Autodesk Inventor part; units mm, degrees
(part 2 of 2)
sketch "スケッチ14" plane through (-202, -25, 10) normal (-1, 0, 0) x (0, 0, 1)
  line L0 (48, 4) -> (0, 4) projected
  line L1 (0, 0) -> (0, 4) projected
  line L2 (0, 0) -> (52, 0) projected
  line L3 (52, 50) -> (52, 0) projected
  line L4 (0, 50) -> (52, 50) projected
  line L5 (0, 46) -> (0, 50) projected
  line L6 (0, 46) -> (48, 46) projected
  line L7 (48, 46) -> (48, 4) projected
  line L8 (-13.92, 46) -> (-6.08, 46) projected
  line L9 (-6.08, 46) -> (-10, 32.2801) projected
  line L10 (-10, 32.2801) -> (-13.92, 46) projected
  line L11 (-16, 38.7199) -> (-12.08, 25) projected
  line L12 (-12.08, 25) -> (-16, 11.2801) projected
  line L13 (-16, 11.2801) -> (-16, 38.7199) projected
  line L14 (-13.92, 4) -> (-10, 17.7199) projected
  line L15 (-10, 17.7199) -> (-6.08, 4) projected
  line L16 (-6.08, 4) -> (-13.92, 4) projected
  line L17 (-4, 11.2801) -> (-7.92, 25) projected
  line L18 (-7.92, 25) -> (-4, 38.7199) projected
  line L19 (-4, 38.7199) -> (-4, 11.2801) projected
  line L20 (-20, 0) -> (0, 0) projected
  line L21 (0, 0) -> (0, 50) projected
  line L22 (0, 50) -> (-20, 50) projected
  line L23 (-20, 50) -> (-20, 0) projected
  line L24 (48, 46) -> (27.8284, 46) projected
  line L25 (44.481, 46) -> (24, 27.4342)
  line L26 (24, 27.4342) -> (4.2197, 46)
  line L27 (0, 46) -> (22.1716, 46) projected
  line L28 (48, 46) -> (24.3744, 24.5837)
  line L29 (27.8284, 4) -> (48, 4) projected
  line L30 (0, 27.7082) -> (0, 46) projected
  line L31 (48, 4) -> (0, 46)
  line L32 (48, 4) -> (48, 46) projected
  line L33 (48, 25) -> (37.9142, 25)
  point P0 (-10, 25)
  dimension "d178" = 2
  constraints: 10 end point, 2 point on line, 1 horizontal, 1 midpoint, 1 parallel
  measures "d178" angle of L31 L26
sketch "スケッチ15" plane through (-202, -25, 10) normal (-1, 0, 0) x (0, 0, 1)
  line L0 (48, 4) -> (0, 4) projected
  line L1 (0, 0) -> (0, 4) projected
  line L2 (0, 0) -> (52, 0) projected
  line L3 (52, 50) -> (52, 0) projected
  line L4 (0, 50) -> (52, 50) projected
  line L5 (0, 46) -> (0, 50) projected
  line L6 (0, 46) -> (48, 46) projected
  line L7 (48, 46) -> (48, 4) projected
  line L8 (48, 46) -> (27.8284, 46) projected
  line L9 (44.3624, 46) -> (0, 5.9989)
  line L10 (0, 4) -> (0, 22.2918) projected
  line L11 (48, 45.1716) -> (48, 27) projected
  line L12 (48, 43.894) -> (3.7564, 4)
  line L13 (0, 4) -> (22.1716, 4) projected
  line L14 (48, 4) -> (48, 46) projected
  line L15 (48, 25) -> (41.7662, 25)
  line L16 (44.3624, 4) -> (0, 44.0011)
  line L17 (48, 6.106) -> (3.7564, 46)
  line L18 (18.8547, 27) -> (0, 27)
  line L19 (0, 27) -> (0, 23)
  line L20 (0, 6.7082) -> (0, 43.2918) projected
  line L21 (0, 23) -> (18.8547, 23)
  point P0 (-10, 25)
  dimension "d179" = 4
  dimension "d180" = 4
  constraints: 16 end point, 7 point on line, 4 symmetric about line, 2 horizontal, 1 midpoint, 1 parallel, 1 perpendicular
  measures "d179" distance between parallel lines of L12 L9
  measures "d180" distance of L18.end L19.end
sketch "スケッチ16" plane through (250, -25, 10) normal (0, 0, 1) x (1, 0, 0)
  line L0 (-97.1716, 4) -> (-102.8284, 4) projected
  line L1 (-97.1716, 0) -> (-97.1716, 4) projected
  line L2 (-52.8284, 0) -> (-97.1716, 0) projected
  line L3 (-52.8284, 0) -> (-52.8284, 4) projected
  line L4 (-50, 4) -> (-52.8284, 4) projected
  line L5 (-50, 4) -> (-50, 0) projected
  line L6 (0, 0) -> (-50, 0) projected
  line L7 (0, 50) -> (0, 0) projected
  line L8 (-50, 50) -> (0, 50) projected
  line L9 (-50, 50) -> (-50, 46) projected
  line L10 (-50, 46) -> (-52.8284, 46) projected
  line L11 (-52.8284, 46) -> (-52.8284, 50) projected
  line L12 (-97.1716, 50) -> (-52.8284, 50) projected
  line L13 (-97.1716, 46) -> (-97.1716, 50) projected
  line L14 (-97.1716, 46) -> (-102.8284, 46) projected
  line L15 (-102.8284, 46) -> (-102.8284, 50) projected
  line L16 (-147.1716, 50) -> (-102.8284, 50) projected
  line L17 (-147.1716, 46) -> (-147.1716, 50) projected
  line L18 (-147.1716, 46) -> (-152.8284, 46) projected
  line L19 (-152.8284, 46) -> (-152.8284, 50) projected
  line L20 (-197.1716, 50) -> (-152.8284, 50) projected
  line L21 (-197.1716, 46) -> (-197.1716, 50) projected
  line L22 (-197.1716, 46) -> (-202.8284, 46) projected
  line L23 (-202.8284, 46) -> (-202.8284, 50) projected
  line L24 (-247.1716, 50) -> (-202.8284, 50) projected
  line L25 (-247.1716, 46) -> (-247.1716, 50) projected
  line L26 (-247.1716, 46) -> (-252.8284, 46) projected
  line L27 (-252.8284, 46) -> (-252.8284, 50) projected
  line L28 (-297.1716, 50) -> (-252.8284, 50) projected
  line L29 (-297.1716, 46) -> (-297.1716, 50) projected
  line L30 (-297.1716, 46) -> (-302.8284, 46) projected
  line L31 (-302.8284, 46) -> (-302.8284, 50) projected
  line L32 (-347.1716, 50) -> (-302.8284, 50) projected
  line L33 (-347.1716, 46) -> (-347.1716, 50) projected
  line L34 (-347.1716, 46) -> (-352.8284, 46) projected
  line L35 (-352.8284, 46) -> (-352.8284, 50) projected
  line L36 (-397.1716, 50) -> (-352.8284, 50) projected
  line L37 (-397.1716, 46) -> (-397.1716, 50) projected
  line L38 (-397.1716, 46) -> (-402.8284, 46) projected
  line L39 (-402.8284, 46) -> (-402.8284, 50) projected
  line L40 (-447.1716, 50) -> (-402.8284, 50) projected
  line L41 (-447.1716, 46) -> (-447.1716, 50) projected
  line L42 (-447.1716, 46) -> (-452, 46) projected
  line L43 (-452, 46) -> (-452, 50) projected
  line L44 (-500, 50) -> (-452, 50) projected
  line L45 (-500, 0) -> (-500, 50) projected
  line L46 (-452, 0) -> (-500, 0) projected
  line L47 (-452, 0) -> (-452, 4) projected
  line L48 (-447.1716, 4) -> (-452, 4) projected
  line L49 (-447.1716, 0) -> (-447.1716, 4) projected
  line L50 (-402.8284, 0) -> (-447.1716, 0) projected
  line L51 (-402.8284, 0) -> (-402.8284, 4) projected
  line L52 (-397.1716, 4) -> (-402.8284, 4) projected
  line L53 (-397.1716, 0) -> (-397.1716, 4) projected
  line L54 (-352.8284, 0) -> (-397.1716, 0) projected
  line L55 (-352.8284, 0) -> (-352.8284, 4) projected
  line L56 (-347.1716, 4) -> (-352.8284, 4) projected
  line L57 (-347.1716, 0) -> (-347.1716, 4) projected
  line L58 (-302.8284, 0) -> (-347.1716, 0) projected
  line L59 (-302.8284, 0) -> (-302.8284, 4) projected
  line L60 (-297.1716, 4) -> (-302.8284, 4) projected
  line L61 (-297.1716, 0) -> (-297.1716, 4) projected
  line L62 (-252.8284, 0) -> (-297.1716, 0) projected
  line L63 (-252.8284, 0) -> (-252.8284, 4) projected
  line L64 (-247.1716, 4) -> (-252.8284, 4) projected
  line L65 (-247.1716, 0) -> (-247.1716, 4) projected
  line L66 (-202.8284, 0) -> (-247.1716, 0) projected
  line L67 (-202.8284, 0) -> (-202.8284, 4) projected
  line L68 (-197.1716, 4) -> (-202.8284, 4) projected
  line L69 (-197.1716, 0) -> (-197.1716, 4) projected
  line L70 (-152.8284, 0) -> (-197.1716, 0) projected
  line L71 (-152.8284, 0) -> (-152.8284, 4) projected
  line L72 (-147.1716, 4) -> (-152.8284, 4) projected
  line L73 (-147.1716, 0) -> (-147.1716, 4) projected
  line L74 (-102.8284, 0) -> (-147.1716, 0) projected
  line L75 (-102.8284, 0) -> (-102.8284, 4) projected
  line L76 (-152, 6.7082) -> (-172.0338, 25) projected
  line L77 (-172.0338, 25) -> (-152, 43.2918) projected
  line L78 (-152, 43.2918) -> (-152, 6.7082) projected
  line L79 (-177.9662, 25) -> (-198, 6.7082) projected
  line L80 (-198, 6.7082) -> (-198, 43.2918) projected
  line L81 (-198, 43.2918) -> (-177.9662, 25) projected
  line L82 (-154.9662, 4) -> (-195.0338, 4) projected
  line L83 (-195.0338, 4) -> (-175, 22.2918) projected
  line L84 (-175, 22.2918) -> (-154.9662, 4) projected
  line L85 (-154.9662, 46) -> (-175, 27.7082) projected
  line L86 (-175, 27.7082) -> (-195.0338, 46) projected
  line L87 (-195.0338, 46) -> (-154.9662, 46) projected
  line L88 (-227.9662, 25) -> (-248, 6.7082) projected
  line L89 (-248, 6.7082) -> (-248, 43.2918) projected
  line L90 (-248, 43.2918) -> (-227.9662, 25) projected
  line L91 (-202, 6.7082) -> (-222.0338, 25) projected
  line L92 (-222.0338, 25) -> (-202, 43.2918) projected
  line L93 (-202, 43.2918) -> (-202, 6.7082) projected
  line L94 (-204.9662, 4) -> (-245.0338, 4) projected
  line L95 (-245.0338, 4) -> (-225, 22.2918) projected
  line L96 (-225, 22.2918) -> (-204.9662, 4) projected
  line L97 (-204.9662, 46) -> (-225, 27.7082) projected
  line L98 (-225, 27.7082) -> (-245.0338, 46) projected
  line L99 (-245.0338, 46) -> (-204.9662, 46) projected
  line L100 (-252, 6.7082) -> (-272.0338, 25) projected
  line L101 (-272.0338, 25) -> (-252, 43.2918) projected
  line L102 (-252, 6.7082) -> (-252, 43.2918) projected
  line L103 (-345.0338, 4) -> (-325, 22.2918) projected
  line L104 (-325, 22.2918) -> (-304.9662, 4) projected
  line L105 (-345.0338, 4) -> (-304.9662, 4) projected
  line L106 (-254.9662, 46) -> (-275, 27.7082) projected
  line L107 (-275, 27.7082) -> (-295.0338, 46) projected
  line L108 (-254.9662, 46) -> (-295.0338, 46) projected
  line L109 (-304.9662, 46) -> (-345.0338, 46) projected
  line L110 (-304.9662, 46) -> (-325, 27.7082) projected
  line L111 (-325, 27.7082) -> (-345.0338, 46) projected
  line L112 (-354.9662, 46) -> (-375, 27.7082) projected
  line L113 (-375, 27.7082) -> (-395.0338, 46) projected
  line L114 (-354.9662, 46) -> (-395.0338, 46) projected
  line L115 (-295.0338, 4) -> (-254.9662, 4) projected
  line L116 (-295.0338, 4) -> (-275, 22.2918) projected
  line L117 (-275, 22.2918) -> (-254.9662, 4) projected
  line L118 (-395.0338, 4) -> (-354.9662, 4) projected
  line L119 (-395.0338, 4) -> (-375, 22.2918) projected
  line L120 (-375, 22.2918) -> (-354.9662, 4) projected
  line L121 (-445.0338, 4) -> (-425, 22.2918) projected
  line L122 (-425, 22.2918) -> (-404.9662, 4) projected
  line L123 (-445.0338, 4) -> (-404.9662, 4) projected
  line L124 (-404.9662, 46) -> (-445.0338, 46) projected
  line L125 (-404.9662, 46) -> (-425, 27.7082) projected
  line L126 (-425, 27.7082) -> (-445.0338, 46) projected
  line L127 (-322.0338, 25) -> (-302, 43.2918) projected
  line L128 (-302, 43.2918) -> (-302, 6.7082) projected
  line L129 (-302, 6.7082) -> (-322.0338, 25) projected
  line L130 (-298, 43.2918) -> (-277.9662, 25) projected
  line L131 (-277.9662, 25) -> (-298, 6.7082) projected
  line L132 (-298, 6.7082) -> (-298, 43.2918) projected
  line L133 (-372.0338, 25) -> (-352, 43.2918) projected
  line L134 (-352, 43.2918) -> (-352, 6.7082) projected
  line L135 (-352, 6.7082) -> (-372.0338, 25) projected
  line L136 (-348, 43.2918) -> (-327.9662, 25) projected
  line L137 (-327.9662, 25) -> (-348, 6.7082) projected
  line L138 (-348, 6.7082) -> (-348, 43.2918) projected
  line L139 (-452, 4.8284) -> (-471.6499, 24.4784) projected
  line L140 (-471.6499, 24.4784) -> (-452, 43.2351) projected
  line L141 (-452, 4.8284) -> (-452, 43.2351) projected
  line L142 (-456.8284, 4) -> (-493.1034, 4) projected
  line L143 (-493.1034, 4) -> (-474.5441, 21.7157) projected
  line L144 (-474.5441, 21.7157) -> (-456.8284, 4) projected
  line L145 (-496, 6.7649) -> (-496, 43.1716) projected
  line L146 (-496, 43.1716) -> (-477.3733, 24.5449) projected
  line L147 (-477.3733, 24.5449) -> (-496, 6.7649) projected
  line L148 (-454.8966, 46) -> (-474.4791, 27.3075) projected
  line L149 (-474.4791, 27.3075) -> (-493.1716, 46) projected
  line L150 (-493.1716, 46) -> (-454.8966, 46) projected
  line L151 (-448, 43.2918) -> (-427.9662, 25) projected
  line L152 (-427.9662, 25) -> (-448, 6.7082) projected
  line L153 (-448, 6.7082) -> (-448, 43.2918) projected
  line L154 (-422.0338, 25) -> (-402, 43.2918) projected
  line L155 (-402, 43.2918) -> (-402, 6.7082) projected
  line L156 (-402, 6.7082) -> (-422.0338, 25) projected
  line L157 (-398, 43.2918) -> (-377.9662, 25) projected
  line L158 (-377.9662, 25) -> (-398, 6.7082) projected
  line L159 (-398, 6.7082) -> (-398, 43.2918) projected
  line L160 (-104.9662, 4) -> (-145.0338, 4) projected
  line L161 (-145.0338, 4) -> (-125, 22.2918) projected
  line L162 (-125, 22.2918) -> (-104.9662, 4) projected
  line L163 (-104.9662, 46) -> (-125, 27.7082) projected
  line L164 (-125, 27.7082) -> (-145.0338, 46) projected
  line L165 (-145.0338, 46) -> (-104.9662, 46) projected
  line L166 (-127.9662, 25) -> (-148, 6.7082) projected
  line L167 (-148, 6.7082) -> (-148, 43.2918) projected
  line L168 (-148, 43.2918) -> (-127.9662, 25) projected
  line L169 (-102, 6.7082) -> (-122.0338, 25) projected
  line L170 (-122.0338, 25) -> (-102, 43.2918) projected
  line L171 (-102, 43.2918) -> (-102, 6.7082) projected
  line L172 (-54.9662, 46) -> (-75, 27.7082) projected
  line L173 (-75, 27.7082) -> (-95.0338, 46) projected
  line L174 (-95.0338, 46) -> (-54.9662, 46) projected
  line L175 (-54.9662, 4) -> (-95.0338, 4) projected
  line L176 (-95.0338, 4) -> (-75, 22.2918) projected
  line L177 (-75, 22.2918) -> (-54.9662, 4) projected
  line L178 (-77.9662, 25) -> (-98, 6.7082) projected
  line L179 (-98, 6.7082) -> (-98, 43.2918) projected
  line L180 (-98, 43.2918) -> (-77.9662, 25) projected
  line L181 (-52, 6.7082) -> (-72.0338, 25) projected
  line L182 (-72.0338, 25) -> (-52, 43.2918) projected
  line L183 (-52, 43.2918) -> (-52, 6.7082) projected
  line L184 (-4, 6.7649) -> (-22.6267, 24.5449) projected
  line L185 (-22.6267, 24.5449) -> (-4, 43.1716) projected
  line L186 (-4, 43.1716) -> (-4, 6.7649) projected
  line L187 (-6.8284, 46) -> (-25.5209, 27.3075) projected
  line L188 (-25.5209, 27.3075) -> (-45.1034, 46) projected
  line L189 (-45.1034, 46) -> (-6.8284, 46) projected
  line L190 (-43.1716, 4) -> (-25.4559, 21.7157) projected
  line L191 (-25.4559, 21.7157) -> (-6.8966, 4) projected
  line L192 (-6.8966, 4) -> (-43.1716, 4) projected
  line L193 (-48, 43.2351) -> (-28.3501, 24.4784) projected
  line L194 (-28.3501, 24.4784) -> (-48, 4.8284) projected
  line L195 (-48, 4.8284) -> (-48, 43.2351) projected
  line L196 (-452, 4.8284) -> (-452, 43.2351) projected
  line L197 (-452, 27.0005) -> (-448, 27.0005)
  line L198 (-448, 27.0005) -> (-448, 23.0005)
  line L199 (-448, 23.0005) -> (-452, 23.0005)
  line L200 (-452, 23.0005) -> (-452, 27.0005)
  point P0 (-250, 25)
  dimension "d181" = 4
  dimension "d182" = 4
  constraints: 8 end point, 2 parallel, 1 horizontal, 1 perpendicular, 1 point on line
  measures "d181" distance of L198.end L199.end
  measures "d182" distance of L197.end L198.end
extrude "押し出し24" add sketch "スケッチ16" along normal blind 48 contours L141 L197 L153 L199
pattern_linear "矩形状パターン3" count 9 spacing 50 along (1, 0, 0) of "押し出し24"
sketch "スケッチ17" plane through (250, -25, 10) normal (0, 0, 1) x (1, 0, 0)
  line L0 (-52, 27.0005) -> (-48, 27.0005) projected
  line L1 (-48, 27.0005) -> (-48, 43.2351) projected
  line L2 (-48, 43.2351) -> (-28.3501, 24.4784) projected
  line L3 (-28.3501, 24.4784) -> (-48, 4.8284) projected
  line L4 (-48, 4.8284) -> (-48, 23.0005) projected
  line L5 (-48, 23.0005) -> (-52, 23.0005) projected
  line L6 (-52, 23.0005) -> (-52, 6.7082) projected
  line L7 (-52, 6.7082) -> (-72.0338, 25) projected
  line L8 (-72.0338, 25) -> (-52, 43.2918) projected
  line L9 (-52, 43.2918) -> (-52, 27.0005) projected
  line L10 (-43.1716, 4) -> (-25.4559, 21.7157) projected
  line L11 (-25.4559, 21.7157) -> (-6.8966, 4) projected
  line L12 (-6.8966, 4) -> (-43.1716, 4) projected
  line L13 (-6.8284, 46) -> (-25.5209, 27.3075) projected
  line L14 (-25.5209, 27.3075) -> (-45.1034, 46) projected
  line L15 (-45.1034, 46) -> (-6.8284, 46) projected
  line L16 (-4, 6.7649) -> (-22.6267, 24.5449) projected
  line L17 (-22.6267, 24.5449) -> (-4, 43.1716) projected
  line L18 (-4, 43.1716) -> (-4, 6.7649) projected
  line L19 (-102, 27.0005) -> (-98, 27.0005) projected
  line L20 (-98, 27.0005) -> (-98, 43.2918) projected
  line L21 (-98, 43.2918) -> (-77.9662, 25) projected
  line L22 (-77.9662, 25) -> (-98, 6.7082) projected
  line L23 (-98, 6.7082) -> (-98, 23.0005) projected
  line L24 (-98, 23.0005) -> (-102, 23.0005) projected
  line L25 (-102, 23.0005) -> (-102, 6.7082) projected
  line L26 (-102, 6.7082) -> (-122.0338, 25) projected
  line L27 (-122.0338, 25) -> (-102, 43.2918) projected
  line L28 (-102, 43.2918) -> (-102, 27.0005) projected
  line L29 (-54.9662, 4) -> (-95.0338, 4) projected
  line L30 (-95.0338, 4) -> (-75, 22.2918) projected
  line L31 (-75, 22.2918) -> (-54.9662, 4) projected
  line L32 (-54.9662, 46) -> (-75, 27.7082) projected
  line L33 (-75, 27.7082) -> (-95.0338, 46) projected
  line L34 (-95.0338, 46) -> (-54.9662, 46) projected
  line L35 (-152, 27.0005) -> (-148, 27.0005) projected
  line L36 (-148, 27.0005) -> (-148, 43.2918) projected
  line L37 (-148, 43.2918) -> (-127.9662, 25) projected
  line L38 (-127.9662, 25) -> (-148, 6.7082) projected
  line L39 (-148, 6.7082) -> (-148, 23.0005) projected
  line L40 (-148, 23.0005) -> (-152, 23.0005) projected
  line L41 (-152, 23.0005) -> (-152, 6.7082) projected
  line L42 (-152, 6.7082) -> (-172.0338, 25) projected
  line L43 (-172.0338, 25) -> (-152, 43.2918) projected
  line L44 (-152, 43.2918) -> (-152, 27.0005) projected
  line L45 (-104.9662, 46) -> (-125, 27.7082) projected
  line L46 (-125, 27.7082) -> (-145.0338, 46) projected
  line L47 (-145.0338, 46) -> (-104.9662, 46) projected
  line L48 (-104.9662, 4) -> (-145.0338, 4) projected
  line L49 (-145.0338, 4) -> (-125, 22.2918) projected
  line L50 (-125, 22.2918) -> (-104.9662, 4) projected
  line L51 (-402, 27.0005) -> (-398, 27.0005) projected
  line L52 (-398, 27.0005) -> (-398, 43.2918) projected
  line L53 (-398, 43.2918) -> (-377.9662, 25) projected
  line L54 (-377.9662, 25) -> (-398, 6.7082) projected
  line L55 (-398, 6.7082) -> (-398, 23.0005) projected
  line L56 (-398, 23.0005) -> (-402, 23.0005) projected
  line L57 (-402, 23.0005) -> (-402, 6.7082) projected
  line L58 (-402, 6.7082) -> (-422.0338, 25) projected
  line L59 (-422.0338, 25) -> (-402, 43.2918) projected
  line L60 (-402, 43.2918) -> (-402, 27.0005) projected
  line L61 (-452, 27.0005) -> (-448, 27.0005) projected
  line L62 (-448, 27.0005) -> (-448, 43.2918) projected
  line L63 (-448, 43.2918) -> (-427.9662, 25) projected
  line L64 (-427.9662, 25) -> (-448, 6.7082) projected
  line L65 (-448, 6.7082) -> (-448, 23.0005) projected
  line L66 (-448, 23.0005) -> (-452, 23.0005) projected
  line L67 (-452, 4.8284) -> (-452, 23.0005) projected
  line L68 (-452, 4.8284) -> (-471.6499, 24.4784) projected
  line L69 (-471.6499, 24.4784) -> (-452, 43.2351) projected
  line L70 (-452, 27.0005) -> (-452, 43.2351) projected
  line L71 (-454.8966, 46) -> (-474.4791, 27.3075) projected
  line L72 (-474.4791, 27.3075) -> (-493.1716, 46) projected
  line L73 (-493.1716, 46) -> (-454.8966, 46) projected
  line L74 (-496, 6.7649) -> (-496, 43.1716) projected
  line L75 (-496, 43.1716) -> (-477.3733, 24.5449) projected
  line L76 (-477.3733, 24.5449) -> (-496, 6.7649) projected
  line L77 (-456.8284, 4) -> (-493.1034, 4) projected
  line L78 (-493.1034, 4) -> (-474.5441, 21.7157) projected
  line L79 (-474.5441, 21.7157) -> (-456.8284, 4) projected
  line L80 (-352, 27.0005) -> (-348, 27.0005) projected
  line L81 (-348, 27.0005) -> (-348, 43.2918) projected
  line L82 (-348, 43.2918) -> (-327.9662, 25) projected
  line L83 (-327.9662, 25) -> (-348, 6.7082) projected
  line L84 (-348, 6.7082) -> (-348, 23.0005) projected
  line L85 (-348, 23.0005) -> (-352, 23.0005) projected
  line L86 (-352, 23.0005) -> (-352, 6.7082) projected
  line L87 (-352, 6.7082) -> (-372.0338, 25) projected
  line L88 (-372.0338, 25) -> (-352, 43.2918) projected
  line L89 (-352, 43.2918) -> (-352, 27.0005) projected
  line L90 (-302, 27.0005) -> (-298, 27.0005) projected
  line L91 (-298, 27.0005) -> (-298, 43.2918) projected
  line L92 (-298, 43.2918) -> (-277.9662, 25) projected
  line L93 (-277.9662, 25) -> (-298, 6.7082) projected
  line L94 (-298, 6.7082) -> (-298, 23.0005) projected
  line L95 (-298, 23.0005) -> (-302, 23.0005) projected
  line L96 (-302, 23.0005) -> (-302, 6.7082) projected
  line L97 (-302, 6.7082) -> (-322.0338, 25) projected
  line L98 (-322.0338, 25) -> (-302, 43.2918) projected
  line L99 (-302, 43.2918) -> (-302, 27.0005) projected
  line L100 (-404.9662, 46) -> (-445.0338, 46) projected
  line L101 (-404.9662, 46) -> (-425, 27.7082) projected
  line L102 (-425, 27.7082) -> (-445.0338, 46) projected
  line L103 (-445.0338, 4) -> (-425, 22.2918) projected
  line L104 (-425, 22.2918) -> (-404.9662, 4) projected
  line L105 (-445.0338, 4) -> (-404.9662, 4) projected
  line L106 (-395.0338, 4) -> (-354.9662, 4) projected
  line L107 (-395.0338, 4) -> (-375, 22.2918) projected
  line L108 (-375, 22.2918) -> (-354.9662, 4) projected
  line L109 (-295.0338, 4) -> (-254.9662, 4) projected
  line L110 (-295.0338, 4) -> (-275, 22.2918) projected
  line L111 (-275, 22.2918) -> (-254.9662, 4) projected
  line L112 (-354.9662, 46) -> (-375, 27.7082) projected
  line L113 (-375, 27.7082) -> (-395.0338, 46) projected
  line L114 (-354.9662, 46) -> (-395.0338, 46) projected
  line L115 (-304.9662, 46) -> (-345.0338, 46) projected
  line L116 (-304.9662, 46) -> (-325, 27.7082) projected
  line L117 (-325, 27.7082) -> (-345.0338, 46) projected
  line L118 (-254.9662, 46) -> (-275, 27.7082) projected
  line L119 (-275, 27.7082) -> (-295.0338, 46) projected
  line L120 (-254.9662, 46) -> (-295.0338, 46) projected
  line L121 (-345.0338, 4) -> (-325, 22.2918) projected
  line L122 (-325, 22.2918) -> (-304.9662, 4) projected
  line L123 (-345.0338, 4) -> (-304.9662, 4) projected
  line L124 (-204.9662, 46) -> (-225, 27.7082) projected
  line L125 (-225, 27.7082) -> (-245.0338, 46) projected
  line L126 (-245.0338, 46) -> (-204.9662, 46) projected
  line L127 (-204.9662, 4) -> (-245.0338, 4) projected
  line L128 (-245.0338, 4) -> (-225, 22.2918) projected
  line L129 (-225, 22.2918) -> (-204.9662, 4) projected
  line L130 (-252, 27.0005) -> (-248, 27.0005) projected
  line L131 (-248, 27.0005) -> (-248, 43.2918) projected
  line L132 (-248, 43.2918) -> (-227.9662, 25) projected
  line L133 (-227.9662, 25) -> (-248, 6.7082) projected
  line L134 (-248, 6.7082) -> (-248, 23.0005) projected
  line L135 (-248, 23.0005) -> (-252, 23.0005) projected
  line L136 (-252, 6.7082) -> (-252, 23.0005) projected
  line L137 (-252, 6.7082) -> (-272.0338, 25) projected
  line L138 (-272.0338, 25) -> (-252, 43.2918) projected
  line L139 (-252, 27.0005) -> (-252, 43.2918) projected
  line L140 (-154.9662, 46) -> (-175, 27.7082) projected
  line L141 (-175, 27.7082) -> (-195.0338, 46) projected
  line L142 (-195.0338, 46) -> (-154.9662, 46) projected
  line L143 (-154.9662, 4) -> (-195.0338, 4) projected
  line L144 (-195.0338, 4) -> (-175, 22.2918) projected
  line L145 (-175, 22.2918) -> (-154.9662, 4) projected
  line L146 (-202, 27.0005) -> (-198, 27.0005) projected
  line L147 (-198, 27.0005) -> (-198, 43.2918) projected
  line L148 (-198, 43.2918) -> (-177.9662, 25) projected
  line L149 (-177.9662, 25) -> (-198, 6.7082) projected
  line L150 (-198, 6.7082) -> (-198, 23.0005) projected
  line L151 (-198, 23.0005) -> (-202, 23.0005) projected
  line L152 (-202, 23.0005) -> (-202, 6.7082) projected
  line L153 (-202, 6.7082) -> (-222.0338, 25) projected
  line L154 (-222.0338, 25) -> (-202, 43.2918) projected
  line L155 (-202, 43.2918) -> (-202, 27.0005) projected
  line L156 (-97.1716, 4) -> (-102.8284, 4) projected
  line L157 (-97.1716, 0) -> (-97.1716, 4) projected
  line L158 (-52.8284, 0) -> (-97.1716, 0) projected
  line L159 (-52.8284, 0) -> (-52.8284, 4) projected
  line L160 (-50, 4) -> (-52.8284, 4) projected
  line L161 (-50, 4) -> (-50, 0) projected
  line L162 (0, 0) -> (-50, 0) projected
  line L163 (0, 50) -> (0, 0) projected
  line L164 (-50, 50) -> (0, 50) projected
  line L165 (-50, 50) -> (-50, 46) projected
  line L166 (-50, 46) -> (-52.8284, 46) projected
  line L167 (-52.8284, 46) -> (-52.8284, 50) projected
  line L168 (-97.1716, 50) -> (-52.8284, 50) projected
  line L169 (-97.1716, 46) -> (-97.1716, 50) projected
  line L170 (-97.1716, 46) -> (-102.8284, 46) projected
  line L171 (-102.8284, 46) -> (-102.8284, 50) projected
  line L172 (-147.1716, 50) -> (-102.8284, 50) projected
  line L173 (-147.1716, 46) -> (-147.1716, 50) projected
  line L174 (-147.1716, 46) -> (-152.8284, 46) projected
  line L175 (-152.8284, 46) -> (-152.8284, 50) projected
  line L176 (-197.1716, 50) -> (-152.8284, 50) projected
  line L177 (-197.1716, 46) -> (-197.1716, 50) projected
  line L178 (-197.1716, 46) -> (-202.8284, 46) projected
  line L179 (-202.8284, 46) -> (-202.8284, 50) projected
  line L180 (-247.1716, 50) -> (-202.8284, 50) projected
  line L181 (-247.1716, 46) -> (-247.1716, 50) projected
  line L182 (-247.1716, 46) -> (-252.8284, 46) projected
  line L183 (-252.8284, 46) -> (-252.8284, 50) projected
  line L184 (-297.1716, 50) -> (-252.8284, 50) projected
  line L185 (-297.1716, 46) -> (-297.1716, 50) projected
  line L186 (-297.1716, 46) -> (-302.8284, 46) projected
  line L187 (-302.8284, 46) -> (-302.8284, 50) projected
  line L188 (-347.1716, 50) -> (-302.8284, 50) projected
  line L189 (-347.1716, 46) -> (-347.1716, 50) projected
  line L190 (-347.1716, 46) -> (-352.8284, 46) projected
  line L191 (-352.8284, 46) -> (-352.8284, 50) projected
  line L192 (-397.1716, 50) -> (-352.8284, 50) projected
  line L193 (-397.1716, 46) -> (-397.1716, 50) projected
  line L194 (-397.1716, 46) -> (-402.8284, 46) projected
  line L195 (-402.8284, 46) -> (-402.8284, 50) projected
  line L196 (-447.1716, 50) -> (-402.8284, 50) projected
  line L197 (-447.1716, 46) -> (-447.1716, 50) projected
  line L198 (-447.1716, 46) -> (-452, 46) projected
  line L199 (-452, 46) -> (-452, 50) projected
  line L200 (-500, 50) -> (-452, 50) projected
  line L201 (-500, 0) -> (-500, 50) projected
  line L202 (-452, 0) -> (-500, 0) projected
  line L203 (-452, 0) -> (-452, 4) projected
  line L204 (-447.1716, 4) -> (-452, 4) projected
  line L205 (-447.1716, 0) -> (-447.1716, 4) projected
  line L206 (-402.8284, 0) -> (-447.1716, 0) projected
  line L207 (-402.8284, 0) -> (-402.8284, 4) projected
  line L208 (-397.1716, 4) -> (-402.8284, 4) projected
  line L209 (-397.1716, 0) -> (-397.1716, 4) projected
  line L210 (-352.8284, 0) -> (-397.1716, 0) projected
  line L211 (-352.8284, 0) -> (-352.8284, 4) projected
  line L212 (-347.1716, 4) -> (-352.8284, 4) projected
  line L213 (-347.1716, 0) -> (-347.1716, 4) projected
  line L214 (-302.8284, 0) -> (-347.1716, 0) projected
  line L215 (-302.8284, 0) -> (-302.8284, 4) projected
  line L216 (-297.1716, 4) -> (-302.8284, 4) projected
  line L217 (-297.1716, 0) -> (-297.1716, 4) projected
  line L218 (-252.8284, 0) -> (-297.1716, 0) projected
  line L219 (-252.8284, 0) -> (-252.8284, 4) projected
  line L220 (-247.1716, 4) -> (-252.8284, 4) projected
  line L221 (-247.1716, 0) -> (-247.1716, 4) projected
  line L222 (-202.8284, 0) -> (-247.1716, 0) projected
  line L223 (-202.8284, 0) -> (-202.8284, 4) projected
  line L224 (-197.1716, 4) -> (-202.8284, 4) projected
  line L225 (-197.1716, 0) -> (-197.1716, 4) projected
  line L226 (-152.8284, 0) -> (-197.1716, 0) projected
  line L227 (-152.8284, 0) -> (-152.8284, 4) projected
  line L228 (-147.1716, 4) -> (-152.8284, 4) projected
  line L229 (-147.1716, 0) -> (-147.1716, 4) projected
  line L230 (-102.8284, 0) -> (-147.1716, 0) projected
  line L231 (-102.8284, 0) -> (-102.8284, 4) projected
  line L232 (-452, 27.0005) -> (-452, 43.2351) projected
  line L233 (-452, 38.1245) -> (-448, 38.1245)
  line L234 (-448, 38.1245) -> (-448, 34.1245)
  line L235 (-448, 34.1245) -> (-452, 34.1245)
  line L236 (-452, 34.1245) -> (-452, 38.1245)
  point P0 (-250, 25)
  dimension "d188" = 4
  dimension "d189" = 4
  constraints: 8 end point, 2 parallel, 1 horizontal, 1 perpendicular, 1 point on line
  measures "d188" distance of L234.end L235.end
  measures "d189" distance of L233.end L234.end
extrude "押し出し25" add sketch "スケッチ17" along normal blind 48 contours L70 L233 L62 L235
pattern_linear "矩形状パターン4" count 9 spacing 50 along (1, 0, 0) of "押し出し25"
sketch "スケッチ18" plane through (200, -25, 62) normal (1, 0, 0) x (0, 0, -1)
  line L0 (27, 46) -> (27, 50) projected
  line L1 (52, 4) -> (4, 4) projected
  line L2 (4, 4) -> (4, 23.0005) projected
  line L3 (4, 23.0005) -> (4, 27.0005) projected
  line L4 (4, 27.0005) -> (4, 34.1245) projected
  line L5 (4, 34.1245) -> (4, 38.1245) projected
  line L6 (4, 38.1245) -> (4, 46) projected
  line L7 (4, 46) -> (52, 46) projected
  line L8 (52, 50) -> (52, 46) projected
  line L9 (52, 50) -> (0, 50) projected
  line L10 (0, 0) -> (0, 50) projected
  line L11 (52, 0) -> (0, 0) projected
  line L12 (52, 4) -> (52, 0) projected
  point P0 (62, 25)
extrude "押し出し26" add sketch "スケッチ18" along normal blind 2 contours L7 L6 L5 L4 L3 L2 L1 L12 L11 L10 L9 L0
